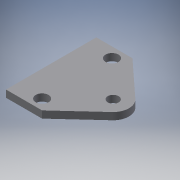
# Autodesk Inventor part: Foundation 6_2
Saved by Autodesk Inventor 2016 (Build 200138000, 138)
## iProperties
Created: 2015-05-27
Part Number: Foundation 6_2
Material: Generic
Document SubType Name: Modeling
Designer: Jonathan
Density: 1 g/cm^3
Appearance: Default
Author: Jonathan
Autodesk Inventor part; units mm, degrees
ref_plane "YZ Plane" through (0, 0, 0) normal (1, 0, 0) x (0, 1, 0)
ref_plane "XZ Plane" through (0, 0, 0) normal (0, 1, 0) x (-1, 0, 0)
ref_plane "XY Plane" through (0, 0, 0) normal (0, 0, 1) x (1, 0, 0)
sketch "Sketch1" plane through (0, 0, 0) normal (0, 1, 0) x (-1, 0, 0)
  line L0 (12.7, -31.75) -> (-12.7, -31.75)
  line L1 (-12.7, -31.75) -> (-12.7, 31.75)
  line L2 (-12.7, 31.75) -> (12.7, 31.75)
  line L3 (12.7, 31.75) -> (12.7, -31.75)
  line L4 (12.7, -31.75) -> (-12.7, 31.75) construction
  line L5 (-12.7, -31.75) -> (12.7, 31.75) construction
  line L6 (-5.5118, -31.75) -> (-5.5118, 31.75)
  line L7 (12.7, 0) -> (-12.7, 0)
  circle A0 centre (-5.5118, 24.5618) radius 3.5052
  circle A1 centre (-5.5118, -24.5618) radius 3.5052
  line L8 (88.6284, 0) -> (-89.1716, 0)
  circle A2 centre (-30.9118, 0) radius 3.81
  line L9 (12.7, 31.75) -> (-12.7, 31.75)
  circle A3 centre (-30.9118, 0) radius 10.9982
  point P0 (0, 0)
  dimension "d0" = 25.4
  dimension "d1" = 63.5
  dimension "d2" = 7.1882
  dimension "d3" = 7.1882
  dimension "d4" = 7.0104
  dimension "d5" = 7.62
  dimension "d6" = 177.8
  dimension "d7" = 0
  dimension "d8" = 25.4
  dimension "d10" = 7.1882
  constraints: 20 end point, 4 centre point, 4 midpoint, 4 point on line, 3 horizontal, 2 parallel, 2 perpendicular, 1 coincident, 1 symmetric about line, 1 other
  measures "d0" distance of L1.end L2.end
  measures "d1" distance of L0.end L1.end
  measures "d2" distance between parallel lines of L1 L6
  measures "d3" distance from line of L2 A0.centre
  measures "d4" diameter of A0
  measures "d5" diameter of A2
  measures "d6" distance of L8.start L8.end
  measures "d7" distance between parallel lines of L7 L8
  measures "d8" distance from line of L6 A2.centre
  measures "d10" radial gap between concentric circles of A3 A2
extrude "Extrusion1" add sketch "Sketch1" along normal blind 5
sketch "Sketch2" plane through (0, 5, 0) normal (0, 1, 0) x (1, 0, 0)
  line L0 (12.7, -31.75) -> (38.3668, -8.086)
  circle A0 centre (30.9118, 0) radius 10.9982 projected
  circle A1 centre (30.9118, 0) radius 10.9982 projected
  line L1 (-12.7, 31.75) -> (-12.7, -31.75) projected
  line L2 (-12.7, 0) -> (12.7, 0)
  line L3 (12.7, -31.75) -> (12.7, 31.75) projected
  line L4 (12.7, 31.75) -> (38.3668, 8.086)
  line L5 (38.3668, 8.086) -> (38.3668, -8.086)
  line L6 (12.7, -31.75) -> (12.7, 31.75)
  point P0 (0, 0)
  constraints: 10 end point, 2 midpoint, 1 parallel, 1 symmetric about line, 1 tangent, 1 vertical, 2 other
extrude "Extrusion2" add sketch "Sketch2" against normal up to surface (5 mm away) contours L3 L4 A0 L0 | A0 L5 picked at (33.4709, -2.7618)
sketch "Sketch3" plane through (0, 5, 0) normal (0, 1, 0) x (1, 0, 0)
  line L0 (12.7, 31.75) -> (12.7, -31.75)
  line L1 (12.7, 31.75) -> (-12.7, 31.75) projected
  line L2 (5.5118, 31.75) -> (5.5118, -31.75)
  line L3 (-12.7, -31.75) -> (12.7, -31.75) projected
  circle A0 centre (5.5118, 24.5618) radius 4.4958
  line L4 (-12.7, 31.75) -> (-12.7, -31.75) projected
  line L5 (-12.7, 0) -> (12.7, 0)
  circle A1 centre (5.5118, -24.5618) radius 4.4958
  circle A2 centre (30.9118, 0) radius 3.81
  point P0 (0, 0)
  dimension "d15" = 7.1882
  dimension "d16" = 7.1882
  dimension "d17" = 8.9916
  dimension "d18" = 25.4
  dimension "d19" = 7.62
  constraints: 6 end point, 3 centre point, 3 point on line, 2 midpoint, 2 vertical, 1 symmetric about line, 1 other
  measures "d15" distance between parallel lines of L0 L2
  measures "d16" distance from line of L1 A0.centre
  measures "d17" diameter of A0
  measures "d18" horizontal distance of A1.centre A2.centre
  measures "d19" diameter of A2
extrude "Extrusion3" cut sketch "Sketch3" against normal through all contours A0 L2 | L2 A0 | A1 L2 | L2 A1 | A2
body "Solid1"
